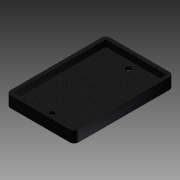
# Autodesk Inventor part: Tapa
Saved by Autodesk Inventor 2016 (Build 200138000, 138)
## iProperties
Created: 2013-07-10
Part Number: Tapa
Material: Generic
Document SubType Name: Modeling
Designer: Luis
Density: 1 g/cm^3
Appearance: Fine Textured - Black
Author: Luis
Autodesk Inventor part; units mm, degrees
ref_plane "YZ Plane" through (0, 0, 0) normal (1, 0, 0) x (0, 1, 0)
ref_plane "XZ Plane" through (0, 0, 0) normal (0, 1, 0) x (-1, 0, 0)
ref_plane "XY Plane" through (0, 0, 0) normal (0, 0, 1) x (1, 0, 0)
sketch "Sketch1" plane through (0, 0, 0) normal (0, 0, 1) x (1, 0, 0)
  circle A0 centre (-1.4563, 20.8) radius 1.5
  circle A1 centre (-1.4563, -20.8) radius 1.5
  arc A2 (-17.4563, 26.8416) -> (-19.7979, 24.5) centre (-17.4563, 24.5) ccw
  line L0 (-19.7979, -24.5) -> (-19.7979, 24.5)
  arc A3 (-19.7979, -24.5) -> (-17.4563, -26.8416) centre (-17.4563, -24.5) ccw
  line L1 (14.5437, -26.8416) -> (-17.4563, -26.8416)
  arc A4 (14.5437, -26.8416) -> (16.8852, -24.5) centre (14.5437, -24.5) ccw
  line L2 (16.8852, 24.5) -> (16.8852, -24.5)
  arc A5 (16.8852, 24.5) -> (14.5437, 26.8416) centre (14.5437, 24.5) ccw
  line L3 (-17.4563, 26.8416) -> (14.5437, 26.8416)
  arc A6 (14.8852, 24.5) -> (14.5437, 24.8416) centre (14.5437, 24.5) ccw
  line L4 (14.8852, 24.5) -> (14.8852, -24.5)
  arc A7 (14.5437, -24.8416) -> (14.8852, -24.5) centre (14.5437, -24.5) ccw
  line L5 (14.5437, -24.8416) -> (-17.4563, -24.8416)
  arc A8 (-17.7979, -24.5) -> (-17.4563, -24.8416) centre (-17.4563, -24.5) ccw
  line L6 (-17.7979, -24.5) -> (-17.7979, 24.5)
  arc A9 (-17.4563, 24.8416) -> (-17.7979, 24.5) centre (-17.4563, 24.5) ccw
  line L7 (-17.4563, 24.8416) -> (14.5437, 24.8416)
  point P0 (0, 0)
  point P1 (0, 0)
  dimension "d0" = 2
  constraints: 16 end point, 16 point on circle, 10 centre point, 7 other
  measures "d0" distance between parallel lines of L3 L7
extrude "Extrusion1" add sketch "Sketch1" along normal blind 6 contours L3 A5 L2 A4 L1 A3 L0 A2
extrude "Extrusion2" add sketch "Sketch1" along normal blind 2.5 contours L4 A7 L5 A8 L6 A9 L7 A6
sketch "Sketch2" plane through (0, 0, 2.5) normal (0, 0, 1) x (1, 0, 0)
  circle A0 centre (-1.4563, -20.8) radius 1.5 projected
  circle A1 centre (-1.4563, 20.8) radius 1.5 projected
  line L0 (14.8852, 24.5) -> (14.8852, -24.5) projected
  arc A2 (14.8852, 24.5) -> (14.5437, 24.8416) centre (14.5437, 24.5) ccw projected
  line L1 (-17.4563, 24.8416) -> (14.5437, 24.8416) projected
  arc A3 (-17.4563, 24.8416) -> (-17.7979, 24.5) centre (-17.4563, 24.5) ccw projected
  line L2 (-17.7979, -24.5) -> (-17.7979, 24.5) projected
  arc A4 (-17.7979, -24.5) -> (-17.4563, -24.8416) centre (-17.4563, -24.5) ccw projected
  line L3 (14.5437, -24.8416) -> (-17.4563, -24.8416) projected
  arc A5 (14.5437, -24.8416) -> (14.8852, -24.5) centre (14.5437, -24.5) ccw projected
  point P0 (0, 0)
chamfer "Chamfer1" distance 1 angle 45 2 edges at (-2.9563, -20.8, 0) (-2.9563, 20.8, 0)
body "Solid1"
